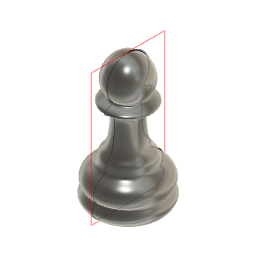
deneyap-piyon-1 v1 (Autodesk Fusion 360 design; units mm, degrees)
Autodesk Fusion 360 part; units mm, degrees
sketch "Sketch1" plane through (0, 0, 0) normal (1, 0, 0) x (0, 1, 0)
  spline S0 degree 5 poles (0.0647, 29.6762) (0.5105, 29.6575) (1.3851, 29.57) (2.6459, 29.2884) (4.2177, 28.6215) (5.9582, 27.3603) (7.4188, 25.7581) (8.5415, 23.9205) (9.2758, 21.9633) (9.5917, 20.0065) (9.4854, 18.1601) (9.0032, 16.5297) (8.2533, 15.2196) (7.4653, 14.2723) (6.9081, 13.6615) (7.1481, 13.1902) (8.4596, 12.6107) (10.0368, 11.9181) (10.9809, 11.1651) (10.7158, 10.4436) (9.6278, 9.7769) (8.1929, 9.102) (6.9262, 8.3064) (6.2046, 7.265) (5.9686, 5.8443) (5.9351, 4.0092) (6.036, 1.8664) (6.2274, -0.4103) (6.5288, -2.6128) (6.9652, -4.5479) (7.5504, -6.0809) (8.2542, -7.1796) (8.9719, -7.9635) (9.5741, -8.6286) (9.9623, -9.361) (10.1234, -10.2578) (10.1837, -11.2365) (10.3536, -12.1565) (10.8482, -12.916) (11.8634, -13.6198) (13.2441, -14.4442) (14.6532, -15.5488) (15.7132, -16.9927) (16.1399, -18.7053) (15.9166, -20.3007) (15.3628, -21.2856) (14.834, -21.7838) (14.6475, -22.0742) (15.0646, -22.7249) (15.8165, -23.741) (16.3938, -24.8348) (16.3799, -25.7794) (15.9193, -26.9366) (15.1161, -28.1703) (14.0533, -29.1774) (12.791, -29.6502) (11.3651, -29.5898) (9.7925, -29.331) (8.0882, -29.0244) (6.2613, -28.8042) (4.3177, -28.7371) (2.6718, -28.8365) (1.3867, -29.002) (0.5075, -29.1528) (0.0622, -29.2383) knots 0 0 0 0 0 0 0.01666667 0.03333333 0.05 0.06666667 0.08333333 0.1 0.11666667 0.13333333 0.15 0.16666667 0.18333333 0.2 0.21666667 0.23333333 0.25 0.26666667 0.28333333 0.3 0.31666667 0.33333333 0.35 0.36666667 0.38333333 0.4 0.41666667 0.43333333 0.45 0.46666667 0.48333333 0.5 0.51666667 0.53333333 0.55 0.56666667 0.58333333 0.6 0.61666667 0.63333333 0.65 0.66666667 0.68333333 0.7 0.71666667 0.73333333 0.75 0.76666667 0.78333333 0.8 0.81666667 0.83333333 0.85 0.86666667 0.88333333 0.9 0.91666667 0.93333333 0.95 0.96666667 0.98333333 1 1 1 1 1 1
  line L0 (-6.9338, 29.9698) -> (7.0632, 29.3825)
  line L1 (9.3394, 26.7398) -> (9.657, 12.7428)
  line L2 (7.1269, 16.392) -> (7.0632, 10.8341)
  line L3 (10.7286, 14.5256) -> (10.7493, 7.3617)
  line L4 (8.235, 12.1262) -> (4.3874, 2.1496)
  line L5 (7.6118, -8.4539) -> (13.805, -16.7448)
  line L6 (15.9523, -11.0837) -> (16.0304, -26.8567)
  line L7 (14.7811, -18.9702) -> (14.7811, -25.1389)
  line L8 (16.3019, -19.5931) -> (16.3428, -31.0733)
  line L9 (18.2168, -28.965) -> (6.8165, -30.1363)
  line L10 (0.0647, 29.6762) -> (0.0622, -29.2383)
  point P0 (9.4982, 19.7413)
  point P1 (7.0951, 13.613)
  point P2 (10.7389, 10.9436)
  point P3 (6.3112, 7.1379)
  point P4 (7.6242, -6.0646)
  point P5 (9.9144, -9.4236)
  point P6 (10.7084, -12.5994)
  point P7 (15.9914, -18.9702)
  point P8 (14.7811, -22.0546)
  point P9 (16.3223, -25.3332)
  point P10 (12.5166, -29.5506)
  constraint midpoint S0.start L0
  constraint midpoint P0 L1
  constraint midpoint P1 L2
  constraint midpoint P2 L3
  constraint midpoint P3 L4
  constraint midpoint P6 L5
  constraint midpoint P7 L6
  constraint midpoint P8 L7
  constraint midpoint P9 L8
  constraint midpoint P10 L9
revolve "Revolve1" add sketch "Sketch1" angle 360 about axis through (0, 0.0647, 29.6762) along (0, -0.000042, -1) contours S0 L6 L10 | S0 L6 picked at (16.0638, -25.6682)
